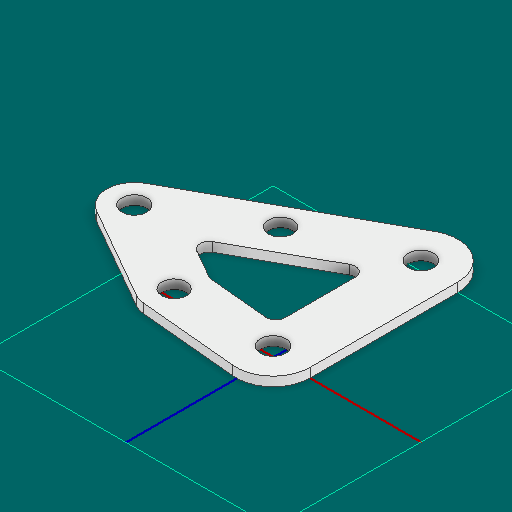
# Autodesk Inventor part: mount
Saved by Autodesk Inventor 2025 (Build 290162000, 162)
## iProperties
Created: 2024-08-21
Part Number: mount
Material: Acetal Resin, White
Document SubType Name: Modeling
Designer: averey
Density: 1.425 g/cm^3
Appearance: Smooth - White
Author: averey
Autodesk Inventor part; units mm, degrees
ref_plane "YZ Plane" through (0, 0, 0) normal (1, 0, 0) x (0, 1, 0)
ref_plane "XZ Plane" through (0, 0, 0) normal (0, 1, 0) x (-1, 0, 0)
ref_plane "XY Plane" through (0, 0, 0) normal (0, 0, 1) x (1, 0, 0)
sketch "main" plane through (0, 0, 0) normal (0, 0, 1) x (1, 0, 0)
  circle A0 centre (15.4343, 10.6591) radius 2.1844
  circle A1 centre (6.35, -22.225) radius 2.15
  circle A2 centre (-9.9657, 10.6591) radius 2.1844
  circle A3 centre (15.4343, -6.35) radius 2.0955
  arc A4 (19.5678, -8.7154) -> (20.176, -6.7945) centre (15.4343, -6.35) ccw
  arc A5 (21.7565, 10.0664) -> (15.4343, 17.0091) centre (15.4343, 10.6591) ccw
  arc A6 (-9.9657, 17.0091) -> (-15.5267, 7.5934) centre (-9.9657, 10.6591) ccw
  arc A7 (2.1793, -24.5243) -> (10.4836, -24.5904) centre (6.35, -22.225) ccw
  line L0 (21.7565, 10.0664) -> (20.176, -6.7945)
  line L1 (15.4343, 17.0091) -> (-9.9657, 17.0091)
  line L2 (-15.5267, 7.5934) -> (2.1793, -24.5243)
  line L3 (19.5678, -8.7154) -> (10.4836, -24.5904)
  line L4 (7.8311, -10.0478) -> (10.6181, -5.1775)
  line L5 (10.8208, -4.5372) -> (11.785, 5.7484)
  line L6 (10.2044, 7.4841) -> (-1.902, 7.4841)
  line L7 (-3.2922, 5.1301) -> (5.063, -10.0258)
  arc A8 (10.6181, -5.1775) -> (10.8208, -4.5372) centre (9.2402, -4.389) ccw
  arc A9 (5.063, -10.0258) -> (7.8311, -10.0478) centre (6.4532, -9.2594) ccw
  arc A10 (-1.902, 7.4841) -> (-3.2922, 5.1301) centre (-1.902, 5.8966) ccw
  arc A11 (11.785, 5.7484) -> (10.2044, 7.4841) centre (10.2044, 5.8966) ccw
  circle A12 centre (-2.909, -6.39) radius 2.0955
  point P0 (7.047, 1.8005)
  dimension "d0" = 4.191
  dimension "d1" = 12.7
  dimension "d2" = 12.7
  dimension "d3" = 9.525
  dimension "d4" = 9.525
  dimension "d5" = 1.5875
  dimension "d8" = 4.7625
  dimension "d9" = 4.191
  measures "d0" diameter of A3
  measures "d1" diameter of A6
  measures "d2" diameter of A5
  measures "d3" diameter of A7
  measures "d4" distance between parallel lines of L3 L4
  measures "d5" radius of A8
  measures "d8" radius of A4
  measures "d9" diameter of A12
sketch "Sketch1" plane through (0, 0, 0) normal (0, 1, 0) x (-1, 0, 0)
  circle A0 centre (0, 0) radius 2.1844
  circle A1 centre (32.891, -9.0591) radius 2.15
  circle A2 centre (0.0195, -25.4) radius 2.1844
  circle A3 centre (17.0091, 0.013) radius 2.0955
  arc A4 (19.3713, 4.1484) -> (17.4499, 4.7551) centre (17.0091, 0.013) ccw
  arc A5 (0.5878, 6.3227) -> (-6.35, -0.0049) centre (0, 0) ccw
  arc A6 (-6.3305, -25.4049) -> (3.0894, -30.9586) centre (0.0195, -25.4) ccw
  arc A7 (35.1935, -13.228) -> (35.2532, -4.9237) centre (32.891, -9.0591) ccw
  line L0 (0.5878, 6.3227) -> (17.4499, 4.7551)
  line L1 (-6.35, -0.0049) -> (-6.3305, -25.4049)
  line L2 (3.0894, -30.9586) -> (35.1935, -13.228)
  line L3 (19.3713, 4.1484) -> (35.2532, -4.9237)
  line L4 (20.7127, -7.5873) -> (15.8402, -4.804)
  line L5 (15.1998, -4.6018) -> (4.9135, -3.6455)
  line L6 (3.179, -5.2274) -> (3.1883, -17.3338)
  line L7 (5.5433, -18.7222) -> (20.6928, -10.3554)
  arc A8 (15.8402, -4.804) -> (15.1998, -4.6018) centre (15.0528, -6.1825) ccw
  arc A9 (20.6928, -10.3554) -> (20.7127, -7.5873) centre (19.9253, -8.9657) ccw
  arc A10 (3.1883, -17.3338) -> (5.5433, -18.7222) centre (4.7758, -17.3326) ccw
  arc A11 (4.9135, -3.6455) -> (3.179, -5.2274) centre (4.7665, -5.2262) ccw
  circle A12 centre (17.0631, -18.3302) radius 2.0955
  point P0 (0, 0)
  constraints: 1 other
extrude "Extrusion1" add sketch "Sketch1" along normal blind 1.5875
body "Solid1"
